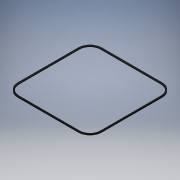
# Autodesk Inventor part: Belt
Saved by Autodesk Inventor 2019 (Build 230136000, 136)
## iProperties
Created: 2017-01-18
Part Number: Belt
Document SubType Name: Modeling
Designer: Administrator
Density: 1 g/cm^3
Mass: 0.541836 g
Surface Area: 17.4488 cm^2
Volume: 0.541836 cm^3
Material: Generic
Appearance: Glossy - Black
Author: Administrator
Autodesk Inventor part; units mm, degrees
ref_plane "YZ Plane" through (0, 0, 0) normal (1, 0, 0) x (0, 1, 0)
ref_plane "XZ Plane" through (0, 0, 0) normal (0, 1, 0) x (-1, 0, 0)
ref_plane "XY Plane" through (0, 0, 0) normal (0, 0, 1) x (1, 0, 0)
sketch "Sketch1" plane through (0, 0, 0) normal (0, 0, 1) x (1, 0, 0)
  line L0 (0, 0) -> (0, 7.5) construction
  line L1 (10, 0) -> (0, 0) construction
  line L2 (0, 0) -> (-10, 0) construction
  line L3 (0, 0) -> (-31.8198, 31.8198) construction
  circle A0 centre (0, 0) radius 45 construction
  line L4 (0, 0) -> (0, 45) construction
  line L5 (-31.8198, 31.8198) -> (-31.8198, -24.2384) construction
  line L6 (-31.8198, -24.2384) -> (-31.8198, -31.8198) construction
  line L7 (-31.8198, 31.8198) -> (24.2384, 31.8198) construction
  line L8 (24.2384, 31.8198) -> (31.8198, 31.8198) construction
  line L9 (31.8198, 31.8198) -> (31.8198, -31.8198) construction
  line L10 (31.8198, -31.8198) -> (-31.8198, -31.8198) construction
  line L11 (0, 0) -> (39.9999, 0) construction
  line L12 (0, 0) -> (0, -40) construction
  line L13 (-31.8198, 44.3198) -> (0, 44.3198)
  line L14 (-44.3198, 31.8198) -> (-44.3198, 0)
  line L15 (-44.3198, 0) -> (0, 0) construction
  arc A1 (-31.8198, 44.3198) -> (-44.3198, 31.8198) centre (-31.8198, 31.8198) ccw
  point P0 (0, 50)
  dimension "d6" = 90
  dimension "d7" = 45
  dimension "d15" = 12.5
  constraints: 32 end point, 7 point on circle, 6 perpendicular, 5 coincident, 3 point on line, 2 centre point, 2 collinear, 2 parallel, 2 tangent, 1 vertical, 2 other
  measures "d6" diameter of A0
  measures "d7" angle of L4 L3
  measures "d15" radius of A1
sketch "Sketch2" plane through (0, 0, 0) normal (1, 0, 0) x (0, 1, 0)
  line L0 (44.3198, 0) -> (44.3198, 0.75)
  line L1 (44.3198, 0.75) -> (42.8198, 0.3481)
  line L2 (42.8198, 0.3481) -> (42.8198, 0)
  line L3 (44.3198, 0) -> (42.8198, 0) construction
  line L4 (44.3198, 0) -> (44.3198, -0.75)
  line L5 (44.3198, -0.75) -> (42.8198, -0.3481)
  line L6 (42.8198, -0.3481) -> (42.8198, 0)
  dimension "d16" = 0.75
  dimension "d17" = 15
  dimension "d18" = 1.5
  constraints: 14 end point, 2 symmetric about line, 1 parallel, 1 perpendicular, 1 vertical
  measures "d16" distance of L0.start L0.end
  measures "d17" angle of L1 L3
  measures "d18" distance between parallel lines of L2 L0
sweep "Sweep1" add profiles "Sketch2" path "Sketch1"
mirror "Mirror1" about plane through (0, 43.6835, 0) normal (1, 0, 0) of "Sweep1"
mirror "Mirror2" about plane through (-44.3198, 0, 0) normal (0, -1, 0) of "Sweep1", "Mirror1"
body "Solid1"
